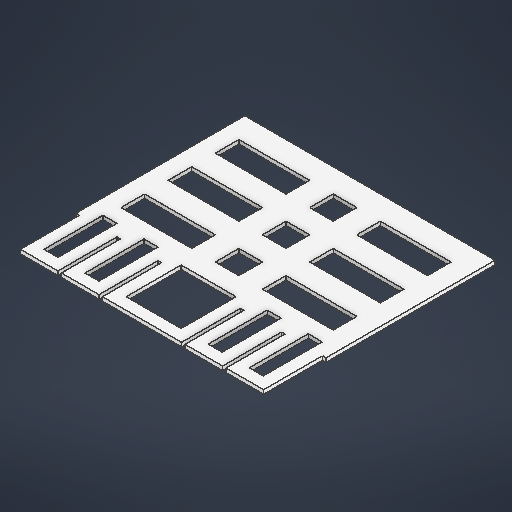
# Autodesk Inventor part: backrest
Saved by Autodesk Inventor 2027.1 (Build 311270010, 270A)
## iProperties
Created: 2025-09-12
Part Number: backrest
Material: Foam Core Board
Document SubType Name: Modeling
Designer: Nick
Density: 0.141998 g/cm^3
Appearance: Default(1)
Mass: 43.462 g
Surface Area: 1456.25 cm^2
Volume: 306.075 cm^3
Author: Nick
Autodesk Inventor part; units mm, degrees
ref_plane "YZ Plane" through (0, 0, 0) normal (1, 0, 0) x (0, 1, 0)
ref_plane "XZ Plane" through (0, 0, 0) normal (0, 1, 0) x (-1, 0, 0)
ref_plane "XY Plane" through (0, 0, 0) normal (0, 0, 1) x (1, 0, 0)
sketch "Sketch1" plane through (0, 0, 0) normal (0, 1, 0) x (-1, 0, 0)
  line L0 (0, 0) -> (318.5, 0)
  line L1 (318.5, 0) -> (318.5, -290)
  line L2 (318.5, -290) -> (0, -290)
  line L3 (0, -290) -> (0, 0)
  dimension "d0" = 318.5
  dimension "d1" = 290
  constraints: 8 end point, 2 parallel, 1 horizontal, 1 perpendicular
  measures "d0" distance of L1.end L2.end
  measures "d1" distance of L0.end L1.end
extrude "Extrusion1" add sketch "Sketch1" along normal blind 5
sketch "Sketch2" plane through (0, 5, 0) normal (0, 1, 0) x (1, 0, 0)
  line L0 (0, 290) -> (-318.5, 290) projected
  line L1 (-318.5, 290) -> (-318.5, 75)
  line L2 (-318.5, 290) -> (-318.5, 0) projected
  line L3 (-318.5, 0) -> (0, 0) projected
  line L4 (-318.5, 75) -> (-314, 75)
  line L5 (-314, 75) -> (-314, 0)
  line L6 (-314, 0) -> (-318.5, 0)
  line L7 (-318.5, 0) -> (-318.5, 75)
  line L8 (-314, 75) -> (-266.25, 75)
  line L9 (-266.25, 75) -> (-261.75, 75)
  line L10 (-261.75, 75) -> (-261.75, 0)
  line L11 (-261.75, 0) -> (-266.25, 0)
  line L12 (-266.25, 0) -> (-266.25, 75)
  line L13 (-261.75, 75) -> (-214, 75)
  line L14 (-214, 75) -> (-209.5, 75)
  line L15 (-209.5, 75) -> (-209.5, 0)
  line L16 (-209.5, 0) -> (-214, 0)
  line L17 (-214, 0) -> (-214, 75)
  line L18 (-209.5, 75) -> (-162.03, 75)
  line L19 (-159.25, 290) -> (-159.25, 0)
  line L20 (0, 75) -> (-4.5, 75)
  line L21 (-4.5, 75) -> (-4.5, 0)
  line L22 (-4.5, 0) -> (0, 0)
  line L23 (0, 0) -> (0, 75)
  line L24 (-4.5, 75) -> (-52.25, 75)
  line L25 (-52.25, 75) -> (-56.75, 75)
  line L26 (-56.75, 75) -> (-56.75, 0)
  line L27 (-56.75, 0) -> (-52.25, 0)
  line L28 (-52.25, 0) -> (-52.25, 75)
  line L29 (-56.75, 75) -> (-104.5, 75)
  line L30 (-104.5, 75) -> (-109, 75)
  line L31 (-109, 75) -> (-109, 0)
  line L32 (-109, 0) -> (-104.5, 0)
  line L33 (-104.5, 0) -> (-104.5, 75)
  point P0 (-214, 0)
  point P1 (-266.25, 0)
  dimension "d4" = 215
  dimension "d5" = 4.5
  dimension "d6" = 47.75
  dimension "d7" = 4.5
  dimension "d8" = 47.75
  dimension "d9" = 4.5
  dimension "d10" = 47.47
  constraints: 62 end point, 13 symmetric about line, 6 parallel, 5 horizontal, 4 perpendicular, 4 point on line, 2 midpoint
  measures "d4" distance of L0.end L1.end
  measures "d5" distance of L5.end L6.end
  measures "d6" distance of L4.end L8.end
  measures "d7" distance of L10.end L11.end
  measures "d8" distance of L9.end L13.end
  measures "d9" distance of L15.end L16.end
  measures "d10" distance of L14.end L18.end
extrude "Extrusion2" cut sketch "Sketch2" against normal blind 5 contours L31 L30 L33 L3 | L4 L5 L3 L2 | L3 L17 L14 L15 | L9 L10 L3 L12 | L26 L25 L28 L3 | L21 L20 L23 L3
sketch "Sketch3" plane through (0, 5, 0) normal (0, 1, 0) x (1, 0, 0)
  line L0 (-318.5, 290) -> (-318.5, 75) projected
  line L1 (-318.5, 290) -> (-296, 290)
  line L2 (-296, 290) -> (-296, 260)
  line L3 (-296, 260) -> (-318.5, 260)
  line L4 (-318.5, 260) -> (-318.5, 290)
  line L5 (-296, 260) -> (-266, 260)
  line L6 (-266, 260) -> (-266, 230)
  line L7 (-266, 230) -> (-296, 230)
  line L8 (-296, 230) -> (-296, 260)
  line L9 (-266, 200) -> (-266, 170)
  line L10 (-266, 170) -> (-296, 170)
  line L11 (-296, 170) -> (-296, 200)
  line L12 (-296, 200) -> (-266, 200)
  line L13 (-266, 140) -> (-266, 110)
  line L14 (-266, 110) -> (-296, 110)
  line L15 (-296, 110) -> (-296, 140)
  line L16 (-296, 140) -> (-266, 140)
  line L17 (-206, 260) -> (-206, 230)
  line L18 (-206, 230) -> (-236, 230)
  line L19 (-236, 230) -> (-236, 260)
  line L20 (-236, 260) -> (-206, 260)
  line L21 (-206, 200) -> (-206, 170)
  line L22 (-206, 170) -> (-236, 170)
  line L23 (-236, 170) -> (-236, 200)
  line L24 (-236, 200) -> (-206, 200)
  line L25 (-206, 140) -> (-206, 110)
  line L26 (-206, 110) -> (-236, 110)
  line L27 (-236, 110) -> (-236, 140)
  line L28 (-236, 140) -> (-206, 140)
  line L29 (-146, 260) -> (-146, 230)
  line L30 (-146, 230) -> (-176, 230)
  line L31 (-176, 230) -> (-176, 260)
  line L32 (-176, 260) -> (-146, 260)
  line L33 (-146, 200) -> (-146, 170)
  line L34 (-146, 170) -> (-176, 170)
  line L35 (-176, 170) -> (-176, 200)
  line L36 (-176, 200) -> (-146, 200)
  line L37 (-146, 140) -> (-146, 110)
  line L38 (-146, 110) -> (-176, 110)
  line L39 (-176, 110) -> (-176, 140)
  line L40 (-176, 140) -> (-146, 140)
  line L41 (-86, 260) -> (-86, 230)
  line L42 (-86, 230) -> (-116, 230)
  line L43 (-116, 230) -> (-116, 260)
  line L44 (-116, 260) -> (-86, 260)
  line L45 (-86, 200) -> (-86, 170)
  line L46 (-86, 170) -> (-116, 170)
  line L47 (-116, 170) -> (-116, 200)
  line L48 (-116, 200) -> (-86, 200)
  line L49 (-86, 140) -> (-86, 110)
  line L50 (-86, 110) -> (-116, 110)
  line L51 (-116, 110) -> (-116, 140)
  line L52 (-116, 140) -> (-86, 140)
  line L53 (-26, 260) -> (-26, 230)
  line L54 (-26, 230) -> (-56, 230)
  line L55 (-56, 230) -> (-56, 260)
  line L56 (-56, 260) -> (-26, 260)
  line L57 (-26, 200) -> (-26, 170)
  line L58 (-26, 170) -> (-56, 170)
  line L59 (-56, 170) -> (-56, 200)
  line L60 (-56, 200) -> (-26, 200)
  line L61 (-26, 140) -> (-26, 110)
  line L62 (-26, 110) -> (-56, 110)
  line L63 (-56, 110) -> (-56, 140)
  line L64 (-56, 140) -> (-26, 140)
  line L65 (-266, 200) -> (-236, 200)
  line L66 (-236, 200) -> (-236, 170)
  line L67 (-236, 170) -> (-266, 170)
  line L68 (-266, 170) -> (-266, 200)
  line L69 (-86, 200) -> (-56, 200)
  line L70 (-56, 200) -> (-56, 170)
  line L71 (-56, 170) -> (-86, 170)
  line L72 (-86, 170) -> (-86, 200)
  line L73 (-86, 260) -> (-56, 260)
  line L74 (-56, 260) -> (-56, 230)
  line L75 (-56, 230) -> (-86, 230)
  line L76 (-86, 230) -> (-86, 260)
  line L77 (-266, 260) -> (-236, 260)
  line L78 (-236, 260) -> (-236, 230)
  line L79 (-236, 230) -> (-266, 230)
  line L80 (-266, 230) -> (-266, 260)
  line L81 (-266, 140) -> (-236, 140)
  line L82 (-236, 140) -> (-236, 110)
  line L83 (-236, 110) -> (-266, 110)
  line L84 (-266, 110) -> (-266, 140)
  line L85 (-86, 140) -> (-56, 140)
  line L86 (-56, 140) -> (-56, 110)
  line L87 (-56, 110) -> (-86, 110)
  line L88 (-86, 110) -> (-86, 140)
  line L89 (-209.5, 0) -> (-109, 0) projected
  line L90 (-209.5, 0) -> (-194.5, 0)
  line L91 (-194.5, 0) -> (-194.5, 15)
  line L92 (-194.5, 15) -> (-209.5, 15)
  line L93 (-209.5, 15) -> (-209.5, 0)
  line L94 (-194.5, 15) -> (-124.5, 15)
  line L95 (-124.5, 15) -> (-124.5, 85)
  line L96 (-124.5, 85) -> (-194.5, 85)
  line L97 (-194.5, 85) -> (-194.5, 15)
  line L98 (-314, 0) -> (-314, 75) projected
  line L99 (-314, 0) -> (-299, 0)
  line L100 (-299, 0) -> (-299, 15)
  line L101 (-299, 15) -> (-314, 15)
  line L102 (-314, 15) -> (-314, 0)
  line L103 (-266.25, 75) -> (-266.25, 0) projected
  line L104 (-266.25, 75) -> (-281.25, 75)
  line L105 (-281.25, 75) -> (-281.25, 90)
  line L106 (-281.25, 90) -> (-266.25, 90)
  line L107 (-266.25, 90) -> (-266.25, 75)
  line L108 (-281.25, 90) -> (-299, 90)
  line L109 (-299, 90) -> (-299, 15)
  line L110 (-299, 15) -> (-281.25, 15)
  line L111 (-281.25, 15) -> (-281.25, 90)
  line L112 (-229, 15) -> (-229, 90)
  line L113 (-246.75, 90) -> (-246.75, 15)
  line L114 (-246.75, 15) -> (-229, 15)
  line L115 (-229, 90) -> (-246.75, 90)
  line L116 (-176.75, 15) -> (-176.75, 90)
  line L117 (-194.5, 90) -> (-194.5, 15)
  line L118 (-194.5, 15) -> (-176.75, 15)
  line L119 (-176.75, 90) -> (-194.5, 90)
  line L120 (-124.5, 15) -> (-124.5, 90)
  line L121 (-142.25, 90) -> (-142.25, 15)
  line L122 (-142.25, 15) -> (-124.5, 15)
  line L123 (-124.5, 90) -> (-142.25, 90)
  line L124 (-72.25, 15) -> (-72.25, 90)
  line L125 (-90, 90) -> (-90, 15)
  line L126 (-90, 15) -> (-72.25, 15)
  line L127 (-72.25, 90) -> (-90, 90)
  line L128 (-20, 15) -> (-20, 90)
  line L129 (-37.75, 90) -> (-37.75, 15)
  line L130 (-37.75, 15) -> (-20, 15)
  line L131 (-20, 90) -> (-37.75, 90)
  point P0 (-209.5, 75)
  dimension "d25" = 22.5
  dimension "d26" = 30
  dimension "d27" = 30
  dimension "d28" = 30
  dimension "d31" = 60
  dimension "d34" = 60
  dimension "d37" = 15
  dimension "d38" = 15
  dimension "d39" = 70
  dimension "d40" = 70
  dimension "d41" = 15
  dimension "d42" = 15
  dimension "d43" = 15
  dimension "d44" = 15
  dimension "d47" = 52.25
  constraints: 256 end point, 26 parallel, 15 horizontal, 13 perpendicular, 2 collinear, 1 vertical, 150 other
  measures "d25" distance of L2.end L3.end
  measures "d26" distance of L1.end L2.end
  measures "d27" distance of L6.end L7.end
  measures "d28" distance of L5.end L6.end
  measures "d31" distance of L5.end L9.start
  measures "d34" distance of L5.end L17.start
  measures "d37" distance of L92.end L91.end
  measures "d38" distance of L91.end L90.end
  measures "d39" distance of L96.end L95.end
  measures "d40" distance of L95.end L94.end
  measures "d41" distance of L101.end L100.end
  measures "d42" distance of L100.end L99.end
  measures "d43" distance of L105.end L106.end
  measures "d44" distance of L104.end L105.end
  measures "d47" distance of L110.end L112.start
extrude "Extrusion3" cut sketch "Sketch3" against normal blind 5 contours L5 L6 L7 L8 | L77 L19 L79 L6 | L20 L17 L18 L19 | L65 L23 L67 L9 | L9 L10 L11 L12 | L24 L21 L22 L23 | L81 L27 L83 L13 | L13 L14 L15 L16 | L28 L25 L26 L27 | L29 L30 L31 L32 | L33 L34 L35 L36 | L37 L38 L39 L40 | L73 L55 L75 L41 | L41 L42 L43 L44 | L56 L53 L54 L55 | L69 L59 L71 L45 | L45 L46 L47 L48 | L60 L57 L58 L59 | L85 L63 L87 L49 | L49 L50 L51 L52 | L64 L61 L62 L63 | L97 L96 L116 L94 | L116 L96 L121 L94 | L121 L96 L95 L94 | L109 L108 L105 L111 L110 | L114 L113 L115 L112 | L126 L125 L127 L124 | L130 L129 L131 L128
body "Solid1"
